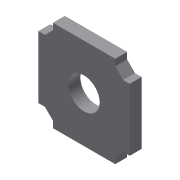
# Autodesk Inventor part: 20_Cube_Insert_Laser_Holder_fixed_v3
Saved by Autodesk Inventor 2019.4 (Build 234330000, 330)
## iProperties
Created: 2019-07-01
Part Number: 20_Cube_Insert_Laser_Holder_fixed_v3
Material: Generic
Document SubType Name: Modeling
Designer: diederichbenedict
Density: 1 g/cm^3
Appearance: Default
Author: diederichbenedict
Autodesk Inventor part; units mm, degrees
ref_plane "YZ Plane" through (0, 0, 0) normal (1, 0, 0) x (0, 1, 0)
ref_plane "Work Plane1" through (0, 0, 10) normal (0, 0, 1) x (1, 0, 0)
sketch "Sketch1" plane through (0, 0, 10) normal (0, 0, 1) x (1, 0, 0)
  line L0 (-4.0299, -0.3538) -> (-2.2322, 1.4439) construction
  arc A0 (-1.4439, 2.2322) -> (-2.2322, 1.4439) centre (-0.9299, 0.9299) ccw construction
  line L1 (-1.4439, 2.2322) -> (0.3538, 4.0299) construction
  line L2 (-37.8299, 42.2137) -> (-37.8299, 45.8299) construction
  line L3 (-37.8299, 45.8299) -> (-4.0299, 45.8299) construction
  line L4 (-4.0299, 45.8299) -> (-4.0299, 42.2137) construction
  line L5 (-4.0299, 4.0299) -> (0.3538, 4.0299) projected
  line L6 (-20.9299, 58.9723) -> (17.1124, 20.9299) construction
  line L7 (17.1124, 20.9299) -> (-20.9299, -17.1124) construction
  line L8 (-20.9299, -17.1124) -> (-58.9723, 20.9299) construction
  line L9 (-58.9723, 20.9299) -> (-20.9299, 58.9723) construction
  line L10 (-20.9299, 58.9723) -> (-20.9299, -17.1124) construction
  line L11 (17.1124, 20.9299) -> (-58.9723, 20.9299) construction
  line L12 (-20.9299, 58.9723) -> (32.8701, 58.9723) construction
  line L13 (-43.4299, 43.4299) -> (1.5701, 43.4299) construction
  line L14 (1.5701, 43.4299) -> (1.5701, -1.5701) construction
  line L15 (1.5701, -1.5701) -> (-43.4299, -1.5701) construction
  line L16 (-43.4299, -1.5701) -> (-43.4299, 43.4299) construction
  line L17 (-43.4299, 43.4299) -> (1.5701, -1.5701) construction
  line L18 (1.5701, 43.4299) -> (-43.4299, -1.5701) construction
  line L19 (-43.4299, 5.3876) -> (-43.4299, 36.4723)
  line L20 (-43.4299, 36.4723) -> (-36.4723, 43.4299)
  line L21 (-36.4723, 43.4299) -> (-5.3876, 43.4299)
  line L22 (-5.3876, 43.4299) -> (1.5701, 36.4723)
  line L23 (1.5701, 36.4723) -> (1.5701, 5.3876)
  line L24 (1.5701, 5.3876) -> (-5.3876, -1.5701)
  line L25 (-5.3876, -1.5701) -> (-36.4723, -1.5701)
  line L26 (-36.4723, -1.5701) -> (-43.4299, 5.3876)
  line L27 (-4.0299, 42.2137) -> (-37.8299, 42.2137) projected
  line L28 (-4.0299, -0.3538) -> (-4.0299, 4.0299) projected
  circle A1 centre (-20.9299, 20.9299) radius 13.3985
  circle A2 centre (-20.9299, 20.9299) radius 15.4895
  point P0 (-37.8299, 4.0299)
  dimension "d18" = 53.8
  dimension "d19" = 45
  dimension "d20" = 53.8
  dimension "d21" = 45
  dimension "d22" = 45
  dimension "d30" = 26.797
  dimension "d36" = 30.979
  constraints: 42 end point, 15 point on line, 4 parallel, 3 midpoint, 3 perpendicular, 2 centre point, 2 coincident, 2 horizontal, 1 equal length
  measures "d18" distance of L6.start L6.end
  measures "d19" angle of L6 L12
  measures "d20" distance of L6.end L7.end
  measures "d21" distance of L14.end L15.end
  measures "d22" distance of L13.end L14.end
  measures "d30" diameter of A1
  measures "d36" diameter of A2
extrude "Extrusion1" add sketch "Sketch1" along normal blind 6.5 contours L28 L24 L25 L26 L19 L20 L27 L22 L23 L5 | L5 L24 L28 | L27 L20 L21 L22 | A1 | A2
ref_plane "Work Plane2" through (-40.9959, 0.8639, 22.2359) normal (0, 0, 1) x (1, 0, 0)
sketch "Sketch3" plane through (0, 0, 10) normal (0, 0, -1) x (-1, 0, 0)
  line L0 (37.8299, -0.4701) -> (37.8299, 4.0299) construction
  line L1 (4.0299, 4.0299) -> (4.0299, -0.4701) construction
  line L2 (37.8299, -0.4701) -> (37.8299, 1.1886) construction
  line L3 (4.0299, -3.9701) -> (4.0299, -0.3538) construction
  line L4 (45.8299, 4.0299) -> (42.2137, 4.0299) construction
  line L5 (-0.3538, 4.0299) -> (-3.9701, 4.0299) construction
  line L6 (-3.9701, 37.8299) -> (-0.3538, 37.8299) construction
  line L7 (4.0299, 42.2137) -> (4.0299, 45.8299) construction
  line L8 (37.8299, 45.8299) -> (37.8299, 42.2137) construction
  line L9 (42.2137, 37.8299) -> (45.8299, 37.8299) construction
  line L10 (37.8299, 37.7299) -> (45.8299, 37.7299)
  line L11 (45.8299, 37.7299) -> (45.8299, 4.1299)
  line L12 (45.8299, 4.1299) -> (37.8299, 4.1299)
  line L13 (37.8299, 4.1299) -> (37.8299, 37.7299)
  line L14 (37.7299, 4.0299) -> (4.1299, 4.0299)
  line L15 (4.1299, 4.0299) -> (4.1299, -3.9701)
  line L16 (4.1299, -3.9701) -> (37.7299, -3.9701)
  line L17 (37.7299, -3.9701) -> (37.7299, 4.0299)
  line L18 (4.0299, 4.1299) -> (-3.9701, 4.1299)
  line L19 (-3.9701, 4.1299) -> (-3.9701, 37.7299)
  line L20 (-3.9701, 37.7299) -> (4.0299, 37.7299)
  line L21 (4.0299, 37.7299) -> (4.0299, 4.1299)
  line L22 (4.1299, 37.8299) -> (37.7299, 37.8299)
  line L23 (37.7299, 37.8299) -> (37.7299, 45.8299)
  line L24 (37.7299, 45.8299) -> (4.1299, 45.8299)
  line L25 (4.1299, 45.8299) -> (4.1299, 37.8299)
  point P0 (0, 0)
  dimension "d23" = 0.1
  dimension "d24" = 0.1
  dimension "d25" = 0.1
  dimension "d26" = 0.1
  dimension "d27" = 0.1
  constraints: 32 end point, 8 parallel, 4 horizontal, 4 perpendicular, 3 point on line
  measures "d23" distance between parallel lines of L8 L23
  measures "d24" distance between parallel lines of L7 L25
  measures "d25" distance between parallel lines of L6 L20
  measures "d26" distance between parallel lines of L5 L18
  measures "d27" distance between parallel lines of L1 L15
extrude "Extrusion3" add sketch "Sketch3" against normal up to surface (6.5 mm away)
sketch "Sketch6" plane through (0, 0, 16.5) normal (0, 0, 1) x (1, 0, 0)
  circle A0 centre (-20.9299, 20.9299) radius 15.4895
  circle A1 centre (-20.9299, 20.9299) radius 11
  line L0 (-45.8299, 4.1299) -> (-45.8299, 37.7299) projected
  line L1 (-4.1299, -3.9701) -> (-37.7299, -3.9701) projected
  line L2 (-37.7299, 45.8299) -> (-4.1299, 45.8299) projected
  point P0 (0, 0)
  point P1 (-45.8299, 20.9299)
  point P2 (-20.9299, -3.9701)
  point P3 (-20.9299, 45.8299)
  dimension "d37" = 22
  dimension "d38" = 30.979
  constraints: 3 midpoint, 2 centre point, 2 vertical alignment, 1 coincident, 1 horizontal alignment
  measures "d37" diameter of A1
  measures "d38" diameter of A0
extrude "Extrusion5" cut sketch "Sketch6" against normal blind 12 contours A1
sketch "Skizze12" plane through (0, 0, 16.5) normal (0, 0, 1) x (1, 0, 0)
  circle A0 centre (-20.9299, 20.9299) radius 11 construction
  line L0 (3.9701, 4.1299) -> (0.3124, 4.1299) projected
  line L1 (3.9701, 37.7299) -> (3.9701, 4.1299) construction
  line L2 (0.3124, 37.7299) -> (3.9701, 37.7299) projected
  line L3 (0.3124, 37.7299) -> (-4.1299, 42.1723) projected
  line L4 (-4.1299, 45.8299) -> (-4.1299, 42.1723) projected
  line L5 (-37.7299, 45.8299) -> (-4.1299, 45.8299) construction
  line L6 (-37.7299, 42.1723) -> (-37.7299, 45.8299) projected
  line L7 (-37.7299, 42.1723) -> (-42.1723, 37.7299) projected
  line L8 (-45.8299, 37.7299) -> (-42.1723, 37.7299) projected
  line L9 (-45.8299, 4.1299) -> (-45.8299, 37.7299) construction
  line L10 (-42.1723, 4.1299) -> (-45.8299, 4.1299) projected
  line L11 (-42.1723, 4.1299) -> (-37.7299, -0.3124) projected
  line L12 (-37.7299, -3.9701) -> (-37.7299, -0.3124) projected
  line L13 (-4.1299, -3.9701) -> (-37.7299, -3.9701) construction
  line L14 (-4.1299, -0.3124) -> (-4.1299, -3.9701) projected
  line L15 (-4.1299, -0.3124) -> (0.3124, 4.1299) projected
  line L16 (-3.9299, 46.0299) -> (-3.9299, 42.2551)
  line L17 (-3.9299, 42.2551) -> (0.3953, 37.9299)
  line L18 (0.3953, 37.9299) -> (4.1701, 37.9299)
  line L19 (4.1701, 37.9299) -> (4.1701, 3.9299) construction
  line L20 (4.1701, 3.9299) -> (0.3953, 3.9299)
  line L21 (0.3953, 3.9299) -> (-3.9299, -0.3953)
  line L22 (-3.9299, -0.3953) -> (-3.9299, -4.1701)
  line L23 (-3.9299, -4.1701) -> (-37.9299, -4.1701) construction
  line L24 (-37.9299, -4.1701) -> (-37.9299, -0.3953)
  line L25 (-37.9299, -0.3953) -> (-42.2551, 3.9299)
  line L26 (-42.2551, 3.9299) -> (-46.0299, 3.9299)
  line L27 (-46.0299, 3.9299) -> (-46.0299, 37.9299) construction
  line L28 (-46.0299, 37.9299) -> (-42.2551, 37.9299)
  line L29 (-42.2551, 37.9299) -> (-37.9299, 42.2551)
  line L30 (-37.9299, 42.2551) -> (-37.9299, 46.0299)
  line L31 (-37.9299, 46.0299) -> (-3.9299, 46.0299) construction
  line L32 (-45.8299, 37.7299) -> (-45.8299, 37.9299)
  line L33 (-37.7299, 45.8299) -> (-37.9299, 45.8299)
  line L34 (-4.1299, 45.8299) -> (-3.9299, 45.8299)
  line L35 (3.9701, 37.7299) -> (3.9701, 37.9299)
  line L36 (3.9701, 4.1299) -> (0.3124, 4.1299) projected
  line L37 (3.9701, 4.1299) -> (3.9701, 3.9299)
  line L38 (-4.1299, -3.9701) -> (-3.9299, -3.9701)
  line L39 (-37.7299, -3.9701) -> (-37.9299, -3.9701)
  line L40 (-45.8299, 4.1299) -> (-45.8299, 3.9299)
  point P0 (0, 0)
  dimension "d93" = 0.2
  constraints: 48 end point, 12 point on line, 4 perpendicular, 15 other
  measures "d93" distance between parallel lines of L5 L31
extrude "IM_offset" add sketch "Skizze12" against normal up to surface (6.5 mm away)
sketch "Sketch13" plane through (0, 0, 10) normal (0, 0, -1) x (-1, 0, 0)
  arc A0 (8.6799, 30.7299) -> (8.6799, 32.7299) centre (8.6799, 31.7299) ccw projected
  arc A1 (33.1799, 32.7299) -> (33.1799, 30.7299) centre (33.1799, 31.7299) ccw projected
  arc A2 (33.1799, 10.7299) -> (33.1799, 8.7299) centre (33.1799, 9.7299) ccw projected
  arc A3 (8.6799, 8.7299) -> (8.6799, 10.7299) centre (8.6799, 9.7299) ccw projected
  circle A4 centre (8.258, 9.7299) radius 0.9
  circle A5 centre (8.258, 31.7299) radius 0.9
  circle A6 centre (33.4928, 31.7299) radius 0.9
  circle A7 centre (33.4928, 9.7299) radius 0.9
  point P0 (0, 0)
  dimension "d96" = 1.8
  dimension "d97" = 1.8
  dimension "d98" = 1.8
  dimension "d99" = 1.8
  constraints: 4 centre point
  measures "d96" diameter of A4
  measures "d97" diameter of A5
  measures "d98" diameter of A6
  measures "d99" diameter of A7
extrude "Extrusion9" cut sketch "Sketch13" against normal blind 10
sketch "Sketch14" plane through (0, 0, 10) normal (0, 0, -1) x (-1, 0, 0)
  circle A0 centre (20.9299, 20.9299) radius 11 projected
  line L0 (29.9299, 32.0648) -> (11.9299, 32.0648)
  line L1 (11.9299, 32.0648) -> (11.9299, 33.5648)
  line L2 (11.9299, 33.5648) -> (29.9299, 33.5648)
  line L3 (29.9299, 33.5648) -> (29.9299, 32.0648)
  line L4 (29.9299, 32.0648) -> (11.9299, 33.5648) construction
  line L5 (11.9299, 32.0648) -> (29.9299, 33.5648) construction
  line L6 (29.9299, 6.9335) -> (11.9299, 6.9335)
  line L7 (11.9299, 6.9335) -> (11.9299, 8.4335)
  line L8 (11.9299, 8.4335) -> (29.9299, 8.4335)
  line L9 (29.9299, 8.4335) -> (29.9299, 6.9335)
  line L10 (29.9299, 6.9335) -> (11.9299, 8.4335) construction
  line L11 (11.9299, 6.9335) -> (29.9299, 8.4335) construction
  line L12 (6.9935, 29.9299) -> (8.4935, 29.9299)
  line L13 (8.4935, 29.9299) -> (8.4935, 11.9299)
  line L14 (8.4935, 11.9299) -> (6.9935, 11.9299)
  line L15 (6.9935, 11.9299) -> (6.9935, 29.9299)
  line L16 (6.9935, 29.9299) -> (8.4935, 11.9299) construction
  line L17 (8.4935, 29.9299) -> (6.9935, 11.9299) construction
  line L18 (33.3254, 29.9299) -> (34.8254, 29.9299)
  line L19 (34.8254, 29.9299) -> (34.8254, 11.9299)
  line L20 (34.8254, 11.9299) -> (33.3254, 11.9299)
  line L21 (33.3254, 11.9299) -> (33.3254, 29.9299)
  line L22 (33.3254, 29.9299) -> (34.8254, 11.9299) construction
  line L23 (34.8254, 29.9299) -> (33.3254, 11.9299) construction
  point P0 (0, 0)
  point P1 (20.9299, 32.8148)
  point P2 (20.9299, 7.6835)
  point P3 (7.7435, 20.9299)
  point P4 (34.0754, 20.9299)
  dimension "d102" = 18
  dimension "d103" = 1.5
  dimension "d104" = 1.5
  dimension "d105" = 1.5
  dimension "d106" = 18
  dimension "d107" = 1.5
  dimension "d108" = 18
  constraints: 48 end point, 8 midpoint, 8 parallel, 4 horizontal, 4 perpendicular, 1 point on line
  measures "d102" distance of L1.end L2.end
  measures "d103" distance of L0.end L1.end
  measures "d104" distance of L6.end L7.end
  measures "d105" distance of L13.end L14.end
  measures "d106" distance of L12.end L13.end
  measures "d107" distance of L19.end L20.end
  measures "d108" distance of L18.end L19.end
extrude "Extrusion10" add sketch "Sketch14" along normal blind 3 contours L0 L1 L2 L3 | L6 L7 L8 L9 | L12 L13 L14 L15 | L18 L19 L20 L21
chamfer "Chamfer1" distance 3 angle 45 4 edges at (-20.9299, 6.9335, 10) (-6.9935, 20.9299, 10) (-20.9299, 33.5648, 10) (-34.8254, 20.9299, 10)
body "Solid1"
